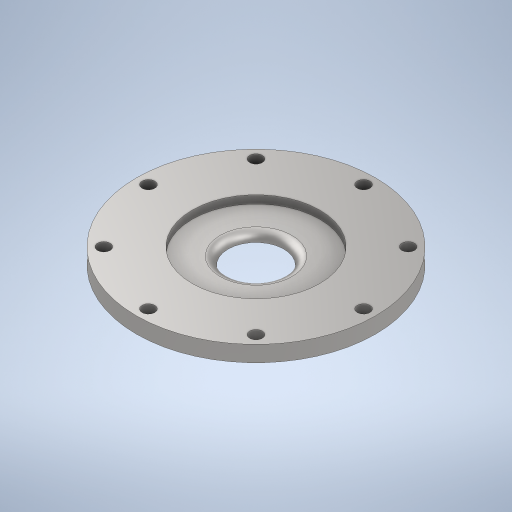
# Autodesk Inventor part: faceplate
Saved by Autodesk Inventor 2023 (Build 270158000, 158)
## iProperties
Created: 2022-07-06
Part Number: faceplate
Material: Stainless Steel
Document SubType Name: Modeling
Designer: pc
Density: 8 g/cm^3
Appearance: Stainless - Brushed
Mass: 1363.93 g
Surface Area: 448.963 cm^2
Volume: 170.491 cm^3
Author: pc
Autodesk Inventor part; units mm, degrees
ref_plane "YZ Plane" through (0, 0, 0) normal (1, 0, 0) x (0, 1, 0)
ref_plane "XZ Plane" through (0, 0, 0) normal (0, 1, 0) x (-1, 0, 0)
ref_plane "XY Plane" through (0, 0, 0) normal (0, 0, 1) x (1, 0, 0)
sketch "Sketch1" plane through (0, 0, 0) normal (0, 1, 0) x (-1, 0, 0)
  circle A0 centre (0, 0) radius 75
  dimension "d0" = 150
  constraints: 1 centre point, 1 coincident
  measures "d0" diameter of A0
extrude "Extrusion1" add sketch "Sketch1" along normal blind 10
sketch "Sketch2" plane through (0, 10, 0) normal (0, 1, 0) x (1, 0, 0)
  circle A0 centre (0, 0) radius 17.5
  dimension "d5" = 35
  constraints: 1 centre point, 1 coincident
  measures "d5" diameter of A0
extrude "Extrusion2" cut sketch "Sketch2" against normal blind 10
sketch "Sketch3" plane through (0, 10, 0) normal (0, 1, 0) x (1, 0, 0)
  circle A0 centre (0, 0) radius 40
  dimension "d8" = 80
  constraints: 1 centre point, 1 coincident
  measures "d8" diameter of A0
extrude "Extrusion3" cut sketch "Sketch3" against normal blind 5
fillet "Fillet2" radius 5 1 edges at (-17.5, 5, 0)
sketch "Sketch5" plane through (0, 10, 0) normal (0, 1, 0) x (1, 0, 0)
  circle A0 centre (0, 0) radius 67.5 construction
  circle A1 centre (0, 67.5) radius 4
  dimension "d46" = 135
  dimension "d47" = 8
  constraints: 1 centre point, 1 coincident, 1 vertical alignment, 2 other
  measures "d47" diameter of A1
hole "Hole2" at (0, 10, -67.5) direction (0, -1, 0) diameter 8 end through all
pattern_circular "Circular Pattern2" count 8 over 360 about axis through (0, -10, 0) along (0, 1, 0) of "Hole2"
body "Solid1"
